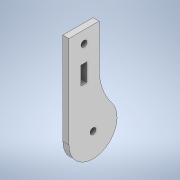
# Autodesk Inventor part: Brazo3Izquierda
Saved by Autodesk Inventor 2022 (Build 260153000, 153)
## iProperties
Created: 2021-09-13
Part Number: Brazo3Izquierda
Material: Generic
Document SubType Name: Modeling
Designer: Administrador
Density: 1 g/cm^3
Appearance: Default
Author: Administrador
Autodesk Inventor part; units mm, degrees
ref_plane "YZ Plane" through (0, 0, 0) normal (1, 0, 0) x (0, 1, 0)
ref_plane "XZ Plane" through (0, 0, 0) normal (0, 1, 0) x (-1, 0, 0)
ref_plane "XY Plane" through (0, 0, 0) normal (0, 0, 1) x (1, 0, 0)
sketch "Sketch1" plane through (0, 0, 0) normal (1, 0, 0) x (0, 1, 0)
  circle A0 centre (0.0036, 0) radius 1.5
  line L0 (-11.9964, 37.6945) -> (46.0036, 37.6945) construction
  line L1 (0.0036, 12) -> (46.0036, 12)
  line L2 (46.0036, 12) -> (46.0036, -3)
  arc A1 (25.9843, -3) -> (7.4266, -9.4286) centre (25.9843, -33) ccw
  line L3 (25.9843, -3) -> (46.0036, -3)
  arc A2 (25.9843, -3) -> (7.4266, -9.4286) centre (25.9843, -33) ccw projected
  line L4 (25.9843, -3) -> (46.0036, -3) projected
  line L5 (46.0036, -3) -> (46.0036, 12) projected
  line L6 (46.0036, 12) -> (0.0036, 12) projected
  circle A3 centre (40.0036, 4.5) radius 1.5 projected
  arc A4 (0.0036, 12) -> (7.4266, -9.4286) centre (0.0036, 0) ccw
  circle A5 centre (40.0036, 4.5) radius 1.5
  line L7 (31.5036, 6) -> (22.5036, 6)
  line L8 (22.5036, 6) -> (22.5036, 3)
  line L9 (22.5036, 3) -> (31.5036, 3)
  line L10 (31.5036, 6) -> (31.5036, 3)
  point P0 (0, 0)
  point P1 (1.5, 26.1095)
  point P2 (22.5, 26.1095)
  dimension "d9" = 58
  dimension "d18" = 9
  dimension "d19" = 3
  dimension "d20" = 6
  dimension "d21" = 7.5
  dimension "d22" = 3
  dimension "d23" = 15
  dimension "d24" = 12
  constraints: 16 end point, 4 centre point, 4 horizontal, 4 point on circle, 2 tangent, 2 vertical, 1 coincident, 1 concentric, 1 parallel, 1 perpendicular
  measures "d9" distance of L0.start L0.end
  measures "d18" distance of L9.end L8.end
  measures "d19" distance of L8.end L7.end
  measures "d20" distance from line of L2 A3.centre
  measures "d21" distance from line of L3 A3.centre
  measures "d22" diameter of A3
  measures "d23" distance between parallel lines of L3 L1
  measures "d24" radius of A4
extrude "Extrusion1" add sketch "Sketch1" along normal blind 3
body "Solid1"
